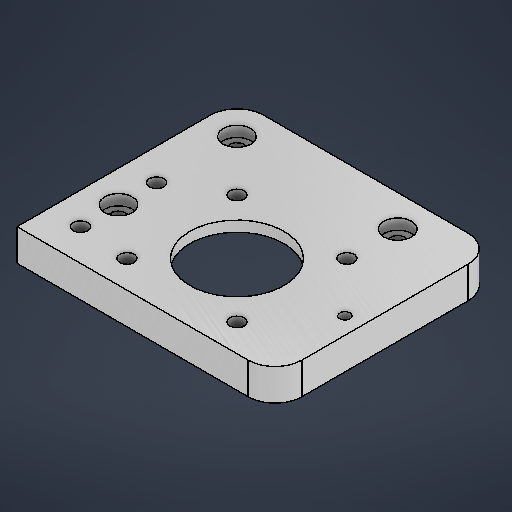
# Autodesk Inventor part: A Drive Frame Lower
Saved by Autodesk Inventor 2026 (Build 300175050, 175E)
## iProperties
Created: 2025-04-15
Part Number: A Drive Frame Lower
Material: Aluminum 6061
Document SubType Name: Modeling
Designer: Joshua Eah
Density: 2.7 g/cm^3
Appearance: Aluminum - Flat
Mass: 51.3122 g
Surface Area: 84.8825 cm^2
Volume: 19.0045 cm^3
Sending System: Autodesk Translation Framework v14.4.0.0
Preprocessor: ST-DEVELOPER v20.1
Title: A Drive Frame Lower.step
Autodesk Inventor part; units mm, degrees
ref_plane "YZ Plane" through (0, 0, 0) normal (1, 0, 0) x (0, 1, 0)
ref_plane "XZ Plane" through (0, 0, 0) normal (0, 1, 0) x (-1, 0, 0)
ref_plane "XY Plane" through (0, 0, 0) normal (0, 0, 1) x (1, 0, 0)
sketch "Main Sketch" plane through (0, 0, 0) normal (0, 1, 0) x (-1, 0, 0)
  line L0 (0, 0) -> (-61, 0)
  line L1 (-61, 0) -> (-61, -52)
  line L2 (-61, -52) -> (0, -52)
  line L3 (0, -52) -> (0, 0)
  circle A0 centre (-7.5, -7.5) radius 1.5
  circle A1 centre (-7.5, -16.5) radius 1.5
  circle A2 centre (-7.5, -25.5) radius 1.5
  circle A3 centre (-19.5, -6.5) radius 1.5
  circle A4 centre (-45.5, -6.5) radius 1.5
  circle A5 centre (-19.5, -32.5) radius 1.5
  circle A6 centre (-45.5, -32.5) radius 1.5
  circle A7 centre (-7.5, -44.5) radius 1.5
  circle A8 centre (-45.5, -44.5) radius 1.5
  circle A9 centre (-57, -20.5) radius 1.5
  circle A10 centre (-32.5, -19.5) radius 11.1125
  dimension "d126" = 61
  dimension "d127" = 52
  dimension "d128" = 3
  dimension "d129" = 7.5
  dimension "d130" = 25.5
  dimension "d131" = 16.5
  dimension "d132" = 7.5
  dimension "d133" = 3
  dimension "d134" = 6.5
  dimension "d135" = 19.5
  dimension "d137" = 45.5
  dimension "d138" = 32.5
  dimension "d139" = 44.5
  dimension "d159" = 57
  dimension "d160" = 20.5
  dimension "d175" = 22.225
  dimension "d176" = 32.5
  dimension "d177" = 19.5
  constraints: 11 centre point, 8 end point, 8 equal radius, 6 vertical alignment, 3 horizontal alignment, 2 parallel, 1 horizontal, 1 perpendicular
  measures "d126" distance of L2.end L1.end
  measures "d127" distance of L2.end L0.start
  measures "d128" diameter of A0
  measures "d129" distance from line of A0.centre L0
  measures "d130" distance from line of A2.centre L0
  measures "d131" distance from line of A1.centre L0
  measures "d132" distance from line of A0.centre L3
  measures "d133" diameter of A3
  measures "d134" distance from line of A3.centre L0
  measures "d135" distance from line of A3.centre L3
  measures "d137" distance from line of A4.centre L3
  measures "d138" distance from line of A5.centre L0
  measures "d139" distance from line of A7.centre L0
  measures "d159" distance from line of A9.centre L3
  measures "d160" distance from line of L0 A9.centre
  measures "d175" diameter of A10
  measures "d176" distance from line of A10.centre L3
  measures "d177" distance from line of A10.centre L0
extrude "Extrusion10" add sketch "Main Sketch" against normal blind 7.5 contours L3 L2 L1 L0 | A0 | A1 | A2 | A3 | A4 | A5 | A6 | A7 | A8 | A9 | A10
hole "Hole14" at (19.5, 0, -32.5) at (45.5, 0, -32.5) at (45.5, 0, -6.5) at (19.5, 0, -6.5) direction (0, -1, 0) diameter 3.4036 end through all clearance for "Socket Head Cap Screw" size "M3" standard "Ansi Metric M Profile"
hole "Frame Mounting Holes" at (7.5, 0, -16.5) at (7.5, 0, -44.5) at (45.5, 0, -44.5) direction (0, -1, 0) diameter 3.4036 end through all counterbore diameter 6.5024 counterbore depth 2.5 clearance for "Socket Head Cap Screw" size "M3" standard "Ansi Metric M Profile"
hole "Hole16" at (57, 0, -20.5) direction (0, -1, 0) diameter 2.459 end through all thread size "M3x0.5" class "6H" standard "ANSI Metric M Profile"
hole "Pin Mounting Holes" at (7.5, 0, -25.5) at (7.5, 0, -7.5) direction (0, -1, 0) diameter 3.4036 depth 5 tip angle 118 clearance for "Socket Head Cap Screw" size "M3" standard "Ansi Metric M Profile"
hole "Hole18" at (32.5, 0, -19.5) direction (0, -1, 0) diameter 22.225 end through all
sketch "Sketch15" plane through (0, -7.5, 0) normal (0, -1, 0) x (1, 0, 0)
  circle A0 centre (32.5, -19.5) radius 11.1125 projected
  circle A1 centre (57, -20.5) radius 1.2295 projected
  circle A2 centre (7.5, -16.5) radius 1.7018 projected
  circle A3 centre (19.5, -6.5) radius 1.7018 projected
  circle A4 centre (45.5, -6.5) radius 1.7018 projected
  circle A5 centre (45.5, -32.5) radius 1.7018 projected
  circle A6 centre (19.5, -32.5) radius 1.7018 projected
  line L0 (61, -52) -> (61, 0) projected
  line L1 (61, 0) -> (0, 0) projected
  line L2 (0, 0) -> (0, -52) projected
  line L3 (0, -52) -> (61, -52) projected
  line L4 (14.8, -1.8) -> (50.2, -1.8)
  line L5 (50.2, -1.8) -> (50.2, -37.2)
  line L6 (50.2, -37.2) -> (14.8, -37.2)
  line L7 (14.8, -37.2) -> (14.8, -1.8)
  dimension "d185" = 14.8
  dimension "d186" = 1.8
  dimension "d187" = 35.4
  dimension "d188" = 35.4
  constraints: 8 end point, 2 parallel, 1 horizontal, 1 perpendicular
  measures "d185" distance between parallel lines of L2 L7
  measures "d186" distance between parallel lines of L1 L4
  measures "d187" distance between parallel lines of L5 L7
  measures "d188" distance of L6.end L4.start
extrude "Extrusion11" cut sketch "Sketch15" against normal blind 5 contours L4 L5 L6 L7
fillet "Fillet1" radius 3.175 4 edges at (14.8, -5, -1.8) (50.2, -5, -1.8) (50.2, -5, -37.2) (14.8, -5, -37.2)
fillet "Fillet2" radius 6.35 3 edges at (61, -3.75, 0) (61, -3.75, -52) (0, -3.75, -52)
equation "\"d131\" = 0.5 * d130 + 0.5 * d129"
body "Solid2"
